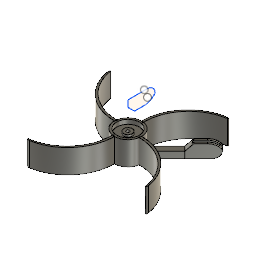
WindSensor_Rotor1 v1 (Autodesk Fusion 360 design; units mm, degrees)
Autodesk Fusion 360 part; units mm, degrees
sketch "Sketch1" plane through (0, 0, 0) normal (1, 0, 0) x (0, 1, 0)
  line L0 (-1.5, 0) -> (0, 1.5)
  line L1 (-1.5, 0) -> (-4, 0)
  line L2 (-4, 0) -> (-4, 2)
  line L3 (-4, 2) -> (-10.5, 2)
  line L4 (-10.5, 2) -> (-10.5, -2)
  line L5 (-10.5, -2) -> (-12.5, -2)
  line L6 (-12.5, -2) -> (-12.5, 20)
  line L7 (-12.5, 20) -> (-1.5, 20)
  line L8 (-1.5, 20) -> (0, 18.5)
  line L9 (0, 18.5) -> (0, 1.5)
  constraint horizontal L1
  constraint perpendicular L1 L2
  constraint perpendicular L2 L3
  constraint perpendicular L3 L4
  constraint perpendicular L4 L5
  constraint perpendicular L5 L6
  constraint perpendicular L6 L7
  constraint perpendicular L7 L9
sketch "Sketch4" plane through (0, 0, 0) normal (0, 0, 1) x (1, 0, 0)
  arc A0 (0, -12.5) -> (36, -55) centre (43.0868, -12.5) ccw
  line L0 (0, -10.5) -> (0, -12.5)
  line L1 (0, -12.5) -> (2, -11.5)
  arc A1 (2, -11.5) -> (38, -54) centre (44.3098, -12.1582) ccw
  arc A2 (36, -55) -> (38.2, -54.8) centre (36.7178, -50.6955) ccw
  arc A3 (38.2, -54.8) -> (38, -54) centre (37.9334, -54.4416) ccw
  point P0 (0, -12.5)
  constraint tangent A0 L0
  constraint coincident P0 A0.start
  constraint tangent A0 A2
  constraint tangent A1 A3
form "Form1" [no effect]
extrude "Extrude1" add sketch "Sketch4" along normal blind 20 makes body 1
form "Form2" [no effect]
revolve "Revolve2" add sketch "Sketch1" angle 360 about axis through (0, 0, 18.5) along (0, 0, -1) separate body makes body 2
move_body "Move1" bodies 1 to x (1, 0, 0) y (0, 1, 0) z (0, 0, 1) at (0, 0, -2)
scale "Scale1" factors (1, 1, 1.1) about (0, -12.5, 18) bodies 1
move_body "Move2" bodies 1 to x (1, 0, 0) y (0, 1, 0) z (0, 0, 1) at (0, 0, 2)
pattern_circular "C-Pattern2" count 4 over 360 about axis through (0, 0, 18.5) along (0, 0, -1) of bodies 1 makes body 3 at (-21.4458, -3.0267, 12.6667) makes body 4 at (-3.0267, 21.4458, 12.6667) makes body 5 at (21.4458, 3.0267, 12.6667)
box "BoxPrimitive1" add length 6 width 61 height 6 placed x (0, -1, 0) y (1, 0, 0) z (0, 0, 1) at (0, 100, 0) separate body makes body 6
move_body "Move3" bodies 6 to x (1, 0, 0) y (0, 1, 0) z (0, 0, 1) at (0, -97.75, 13.25)
move_face "MoveFace1" by (0, 0, 1) 1 faces at (61, -1.75, 15.25) on bodies 6
move_body "Move4" bodies 6 to x (1, 0, 0) y (0, 1, 0) z (0, 0, 1) at (0, 0, 0.5)
move_body "Move5" bodies 6 to x (1, 0, 0) y (0, 1, 0) z (0, 0, 1) at (0, 0, 0.25)
move_body "Move6" bodies 6 to x (1, 0, 0) y (0, 1, 0) z (0, 0, 1) at (0, 0.6, 0)
move_body "Move7" bodies 6 to x (1, 0, 0) y (0, 1, 0) z (0, 0, 1) at (3, 0, 0)
delete_body "RemoveBody1" bodies 6
move_body "Move8" bodies 3 1 2 4 5 to x (1, 0, 0) y (0, 1, 0) z (0, 0, 1) at (0, 0, 2)
move_body "Move9" bodies 3 5 1 4 2 to x (1, 0, 0) y (0, 1, 0) z (0, 0, 1) at (0, 0, -22)
box "BoxPrimitive2" add length 6 width 60 height 6 placed x (0, -1, 0) y (1, 0, 0) z (0, 0, 1) at (-63, 3, 0) separate body makes body 7
move_body "Move10" bodies 7 to x (1, 0, 0) y (0, 1, 0) z (0, 0, 1) at (-2, 0, 0)
copy_body "CopyPasteBodies1" bodies 7 makes body 8
move_body "Move11" bodies 8 to x (1, 0, 0) y (0, 1, 0) z (0, 0, 1) at (70, 0, 0)
move_body "Move12" bodies 8 7 to x (0.707107, -0.707107, 0) y (0.707107, 0.707107, 0) z (0, 0, 1) at (0, 0, 0)
move_body "Move13" bodies 7 8 to x (1, 0, 0) y (0, 1, 0) z (0, 0, 1) at (0, 0, -6)
copy_body "CopyPasteBodies2" bodies 7 makes body 9
delete_body "RemoveBody2" bodies 7
move_face "OffsetFaces1" offset -28 1 faces at (-46.669, 45.2548, -4) on bodies 9
sketch "Sketch7" plane through (0, 0, 0) normal (1, 0, 0) x (0, 1, 0)
  line L0 (0, 45) -> (18, 45)
  line L1 (0, 39) -> (6, 33)
  line L2 (6, 33) -> (15, 33)
  arc A0 (15, 33) -> (25, 38) centre (15, 45.5) ccw
  arc A1 (25, 38) -> (18, 45) centre (18, 38) ccw
  line L3 (0, 45) -> (0, 39)
  constraint horizontal L0
  constraint horizontal L2
  constraint tangent L2 A0
  constraint tangent L0 A1
  constraint perpendicular L0 L3
extrude "Extrude2" add sketch "Sketch7" along normal blind 6 separate body makes body 10
move_body "Move14" bodies 10 to x (0.707107, 0.707107, 0) y (-0.707107, 0.707107, 0) z (0, 0, 1) at (1.7574, -4.2426, 0)
move_body "Move15" bodies 10 to x (1, 0, 0) y (0, 1, 0) z (0, 0, 1) at (-30.0416, 28.2843, -45)
form "Form3" [no effect]
box "BoxPrimitive3" add length 13 width 40 height 2 placed x (0, 0, -1) y (0.707107, -0.707107, 0) z (-0.707107, -0.707107, 0) at (-76.3675, 72.1249, 0) separate body makes body 11
move_body "Move16" bodies 11 to x (1, 0, 0) y (0, 1, 0) z (0, 0, 1) at (2.8284, 2.8284, 0)
move_face "MoveFace2" by (16.2635, -16.2635, 0) 3 faces at (-45.7262, 46.1976, -8.6667) (-55.6257, 55.1543, 0) (-54.6829, 56.0971, -4.3333) on bodies 11
combine "Combine1" operation cut target body 10 tool bodies 11
move_body "Move17" bodies 4 2 10 3 1 9 5 8 to x (-1, 0, 0) y (0, 1, 0) z (0, 0, -1) at (0, 0, 0)
revolve "Revolve1" [suppressed]
